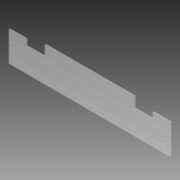
# Autodesk Inventor part: dozer side pannel
Saved by Autodesk Inventor 2012 (Build 160160000, 160)
## iProperties
Created: 2013-10-06
Part Number: dozer side pannel
Material: Default
Document SubType Name: Modeling
Designer: Bryce
Density: 1 g/cm^3
Author: Bryce
Autodesk Inventor part; units mm, degrees
ref_plane "YZ Plane" through (0, 0, 0) normal (1, 0, 0) x (0, 1, 0)
ref_plane "XZ Plane" through (0, 0, 0) normal (0, 1, 0) x (-1, 0, 0)
ref_plane "XY Plane" through (0, 0, 0) normal (0, 0, 1) x (1, 0, 0)
sketch "Sketch1" plane through (0, 0, 0) normal (0, 0, 1) x (1, 0, 0)
  line L0 (0, 0) -> (685.8, 0)
  line L1 (685.8, 0) -> (685.8, 127)
  line L2 (0, 127) -> (0, 0)
  line L3 (152.4, 146.05) -> (152.4, 101.6)
  line L4 (152.4, 101.6) -> (76.2, 101.6)
  line L5 (76.2, 101.6) -> (76.2, 127)
  line L6 (533.4, 146.05) -> (533.4, 101.6)
  line L7 (533.4, 101.6) -> (609.6, 101.6)
  line L8 (609.6, 101.6) -> (609.6, 127)
  line L9 (76.2, 127) -> (0, 127)
  line L10 (685.8, 127) -> (609.6, 127)
  line L11 (533.4, 146.05) -> (152.4, 146.05)
  dimension "d0" = 127
  dimension "d1" = 685.8
  dimension "d4" = 76.2
  dimension "d6" = 76.2
  dimension "d7" = 76.2
  dimension "d8" = 76.2
  dimension "d10" = 25.4
  dimension "d11" = 44.45
  dimension "d12" = 25.4
  constraints: 24 end point, 6 parallel, 3 perpendicular, 1 collinear, 1 horizontal
  measures "d0" distance of L2.start L0.start
  measures "d1" distance of L0.start L0.end
  measures "d4" distance of L3.end L4.end
  measures "d6" distance between parallel lines of L2 L5
  measures "d7" distance between parallel lines of L1 L8
  measures "d8" distance of L6.end L7.end
  measures "d10" distance of L4.end L5.end
  measures "d11" distance of L6.start L6.end
  measures "d12" distance of L7.end L8.end
extrude "Extrusion1" add sketch "Sketch1" along normal blind 6.35
sketch "Sketch2" plane through (685.8, 0, 0) normal (1, 0, 0) x (0, 0, -1)
  line L0 (-6.35, 127) -> (-6.35, 0) projected
  line L1 (0, 0) -> (-6.35, 0) projected
  line L2 (-5.842, 0.508) -> (-0.508, 0.508)
  line L3 (-0.508, 0.508) -> (-0.508, 6.35)
  line L4 (-0.508, 6.35) -> (-5.842, 6.35)
  line L5 (-5.842, 6.35) -> (-5.842, 0.508)
  line L6 (-5.842, 6.8326) -> (-0.508, 6.8326)
  line L7 (-0.508, 6.8326) -> (-0.508, 12.6746)
  line L8 (-0.508, 12.6746) -> (-5.842, 12.6746)
  line L9 (-5.842, 12.6746) -> (-5.842, 6.8326)
  line L10 (-5.842, 13.1572) -> (-0.508, 13.1572)
  line L11 (-0.508, 13.1572) -> (-0.508, 18.9992)
  line L12 (-0.508, 18.9992) -> (-5.842, 18.9992)
  line L13 (-5.842, 18.9992) -> (-5.842, 13.1572)
  line L14 (-5.842, 19.4818) -> (-0.508, 19.4818)
  line L15 (-0.508, 19.4818) -> (-0.508, 25.3238)
  line L16 (-0.508, 25.3238) -> (-5.842, 25.3238)
  line L17 (-5.842, 25.3238) -> (-5.842, 19.4818)
  line L18 (-5.842, 25.8064) -> (-0.508, 25.8064)
  line L19 (-0.508, 25.8064) -> (-0.508, 31.6484)
  line L20 (-0.508, 31.6484) -> (-5.842, 31.6484)
  line L21 (-5.842, 31.6484) -> (-5.842, 25.8064)
  line L22 (-5.842, 32.131) -> (-0.508, 32.131)
  line L23 (-0.508, 32.131) -> (-0.508, 37.973)
  line L24 (-0.508, 37.973) -> (-5.842, 37.973)
  line L25 (-5.842, 37.973) -> (-5.842, 32.131)
  line L26 (-5.842, 38.4556) -> (-0.508, 38.4556)
  line L27 (-0.508, 38.4556) -> (-0.508, 44.2976)
  line L28 (-0.508, 44.2976) -> (-5.842, 44.2976)
  line L29 (-5.842, 44.2976) -> (-5.842, 38.4556)
  line L30 (-5.842, 44.7802) -> (-0.508, 44.7802)
  line L31 (-0.508, 44.7802) -> (-0.508, 50.6222)
  line L32 (-0.508, 50.6222) -> (-5.842, 50.6222)
  line L33 (-5.842, 50.6222) -> (-5.842, 44.7802)
  line L34 (-5.842, 51.1048) -> (-0.508, 51.1048)
  line L35 (-0.508, 51.1048) -> (-0.508, 56.9468)
  line L36 (-0.508, 56.9468) -> (-5.842, 56.9468)
  line L37 (-5.842, 56.9468) -> (-5.842, 51.1048)
  line L38 (-5.842, 57.4294) -> (-0.508, 57.4294)
  line L39 (-0.508, 57.4294) -> (-0.508, 63.2714)
  line L40 (-0.508, 63.2714) -> (-5.842, 63.2714)
  line L41 (-5.842, 63.2714) -> (-5.842, 57.4294)
  line L42 (-5.842, 63.754) -> (-0.508, 63.754)
  line L43 (-0.508, 63.754) -> (-0.508, 69.596)
  line L44 (-0.508, 69.596) -> (-5.842, 69.596)
  line L45 (-5.842, 69.596) -> (-5.842, 63.754)
  line L46 (-5.842, 70.0786) -> (-0.508, 70.0786)
  line L47 (-0.508, 70.0786) -> (-0.508, 75.9206)
  line L48 (-0.508, 75.9206) -> (-5.842, 75.9206)
  line L49 (-5.842, 75.9206) -> (-5.842, 70.0786)
  line L50 (-5.842, 76.4032) -> (-0.508, 76.4032)
  line L51 (-0.508, 76.4032) -> (-0.508, 82.2452)
  line L52 (-0.508, 82.2452) -> (-5.842, 82.2452)
  line L53 (-5.842, 82.2452) -> (-5.842, 76.4032)
  line L54 (-5.842, 82.7278) -> (-0.508, 82.7278)
  line L55 (-0.508, 82.7278) -> (-0.508, 88.5698)
  line L56 (-0.508, 88.5698) -> (-5.842, 88.5698)
  line L57 (-5.842, 88.5698) -> (-5.842, 82.7278)
  line L58 (-5.842, 89.0524) -> (-0.508, 89.0524)
  line L59 (-0.508, 89.0524) -> (-0.508, 94.8944)
  line L60 (-0.508, 94.8944) -> (-5.842, 94.8944)
  line L61 (-5.842, 94.8944) -> (-5.842, 89.0524)
  line L62 (-5.842, 95.377) -> (-0.508, 95.377)
  line L63 (-0.508, 95.377) -> (-0.508, 101.219)
  line L64 (-0.508, 101.219) -> (-5.842, 101.219)
  line L65 (-5.842, 101.219) -> (-5.842, 95.377)
  line L66 (-5.842, 101.7016) -> (-0.508, 101.7016)
  line L67 (-0.508, 101.7016) -> (-0.508, 107.5436)
  line L68 (-0.508, 107.5436) -> (-5.842, 107.5436)
  line L69 (-5.842, 107.5436) -> (-5.842, 101.7016)
  line L70 (-5.842, 108.0262) -> (-0.508, 108.0262)
  line L71 (-0.508, 108.0262) -> (-0.508, 113.8682)
  line L72 (-0.508, 113.8682) -> (-5.842, 113.8682)
  line L73 (-5.842, 113.8682) -> (-5.842, 108.0262)
  line L74 (-5.842, 114.3508) -> (-0.508, 114.3508)
  line L75 (-0.508, 114.3508) -> (-0.508, 120.1928)
  line L76 (-0.508, 120.1928) -> (-5.842, 120.1928)
  line L77 (-5.842, 120.1928) -> (-5.842, 114.3508)
  line L78 (-5.842, 120.6754) -> (-0.508, 120.6754)
  line L79 (-0.508, 120.6754) -> (-0.508, 126.5174)
  line L80 (-0.508, 126.5174) -> (-5.842, 126.5174)
  line L81 (-5.842, 126.5174) -> (-5.842, 120.6754)
  line L82 (-5.842, 127) -> (-0.508, 127)
  line L83 (-0.508, 127) -> (-0.508, 132.842)
  line L84 (-0.508, 132.842) -> (-5.842, 132.842)
  line L85 (-5.842, 132.842) -> (-5.842, 127)
  line L86 (-5.842, 133.3246) -> (-0.508, 133.3246)
  line L87 (-0.508, 133.3246) -> (-0.508, 139.1666)
  line L88 (-0.508, 139.1666) -> (-5.842, 139.1666)
  line L89 (-5.842, 139.1666) -> (-5.842, 133.3246)
  line L90 (-5.842, 139.6492) -> (-0.508, 139.6492)
  line L91 (-0.508, 139.6492) -> (-0.508, 145.4912)
  line L92 (-0.508, 145.4912) -> (-5.842, 145.4912)
  line L93 (-5.842, 145.4912) -> (-5.842, 139.6492)
  dimension "d13" = 5.334
  dimension "d14" = 5.842
  dimension "d15" = 0.508
  dimension "d16" = 0.508
  dimension "d19" = 6.3246
  constraints: 184 end point, 2 parallel, 1 horizontal, 1 perpendicular, 1 vertical, 176 other
  measures "d13" distance of L2.start L2.end
  measures "d14" distance of L4.end L2.start
  measures "d15" distance between parallel lines of L0 L5
  measures "d16" distance between parallel lines of L1 L2
  measures "d19" distance of L2.start L6.start
extrude "Extrusion2" cut sketch "Sketch2" against normal through all
equation "\"d7\" = d6"
equation "\"d8\" = d4"
equation "\"d14\" = d13 + d15"
equation "\"d16\" = d15"
body "Solid1"
